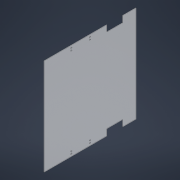
# Autodesk Inventor part: TopV5
Saved by Autodesk Inventor 2022 (Build 260153000, 153)
## iProperties
Created: 2021-10-02
Part Number: TopV5
Material: Acrylic, Clear
Document SubType Name: Sheet Metal
Designer: timmy
Density: 1.19 g/cm^3
Appearance: Transparent - Clear
Sheet Metal Rule: Default
Author: timmy
Autodesk Inventor part; units mm, degrees
ref_plane "YZ Plane" through (0, 0, 0) normal (1, 0, 0) x (0, 1, 0)
ref_plane "XZ Plane" through (0, 0, 0) normal (0, 1, 0) x (-1, 0, 0)
ref_plane "XY Plane" through (0, 0, 0) normal (0, 0, 1) x (1, 0, 0)
sketch "Sketch1" plane through (0, 0, 0) normal (1, 0, 0) x (0, 1, 0)
  line L0 (0, 0) -> (533.4, 0)
  line L1 (533.4, 0) -> (533.4, -508)
  line L2 (533.4, -508) -> (0, -508)
  line L3 (0, -508) -> (0, 0)
  dimension "d0" = 533.4
  dimension "d1" = 508
  constraints: 8 end point, 2 parallel, 1 horizontal, 1 perpendicular
  measures "d0" distance of L1.end L2.end
  measures "d1" distance of L0.end L1.end
extrude "Extrusion1" add sketch "Sketch1" along normal blind 1.5875
sketch "Sketch3" plane through (0, 0, 0) normal (-1, 0, 0) x (0, 0, 1)
  line L0 (-508, 0) -> (-508, 533.4) projected
  line L1 (0, 0) -> (-508, 0) projected
  circle A0 centre (-358.14, 12.7) radius 3.302
  circle A1 centre (-358.14, 25.4) radius 3.302
  circle A2 centre (-149.86, 12.7) radius 3.302
  circle A3 centre (-149.86, 25.4) radius 3.302
  circle A4 centre (-254, 12.7) radius 3.302
  circle A5 centre (-254, 25.4) radius 3.302
  circle A6 centre (-358.14, 508) radius 3.302
  circle A7 centre (-358.14, 520.7) radius 3.302
  circle A8 centre (-149.86, 508) radius 3.302
  circle A9 centre (-149.86, 520.7) radius 3.302
  circle A10 centre (-254, 508) radius 3.302
  circle A11 centre (-254, 520.7) radius 3.302
  constraints: 12 centre point
extrude "Extrusion5" cut sketch "Sketch3" against normal up to surface (1.5875 mm away) contours A0 | A1 | A2 | A3 | A4 | A5
sheet face with bend "Face1" sketch "Sketch1" thickness 3.048 toward (1, 0, 0) bend radius 3.048
bend "Bend1"
extrude "Cut1" cut sketch "Sketch3" against normal up to surface (3.048 mm away)
sketch "Sketch4" plane through (3.048, 0, 0) normal (1, 0, 0) x (0, 0, -1)
  line L0 (508, 533.4) -> (508, 0) projected
  line L1 (508, 266.7) -> (434.34, 266.7)
  line L2 (0, 0) -> (508, 0) projected
  line L3 (434.34, 0) -> (434.34, 34.925)
  line L4 (434.34, 0) -> (469.265, 0) construction
  line L5 (434.34, 34.925) -> (349.377, 34.925)
  line L6 (434.34, 17.4625) -> (346.202, 17.4625)
  line L7 (346.202, 0) -> (346.202, 31.75)
  line L8 (346.202, 31.75) -> (349.377, 34.925)
  line L9 (434.34, 533.4) -> (434.34, 498.475)
  line L10 (434.34, 498.475) -> (349.377, 498.475)
  line L11 (434.34, 515.9375) -> (346.202, 515.9375)
  line L12 (346.202, 533.4) -> (346.202, 501.65)
  line L13 (346.202, 501.65) -> (349.377, 498.475)
  line L14 (0, 533.4) -> (508, 533.4) projected
  line L15 (508, 0) -> (0, 0) projected
  dimension "d42" = 73.66
  dimension "d43" = 34.925
  dimension "d44" = 90
  dimension "d45" = 84.963
  dimension "d46" = 88.138
  dimension "d47" = 31.75
  constraints: 24 end point, 7 symmetric about line, 4 horizontal, 2 midpoint, 2 point on line, 2 vertical, 1 perpendicular
  measures "d42" distance of L1.start L1.end
  measures "d43" distance of L3.start L3.end
  measures "d44" angle of L4 L3
  measures "d45" distance of L3.end L5.end
  measures "d46" distance of L6.start L6.end
  measures "d47" distance of L7.start L7.end
extrude "Cut2" cut sketch "Sketch4" against normal blind 3.048
equation "\"d38\" = Thickness"
equation "\"d48\" = Thickness"
equation "\"d32\" = Thickness"
equation "\"d33\" = BendRadius"
equation "\"d34\" = BendReliefWidth"
equation "\"d36\" = MinimumRemnant"
equation "\"d35\" = BendReliefDepth"
equation "\"d37\" = TransitionRadius"
equation "\"BendRadius\" = Thickness"
equation "\"BendReliefWidth\" = Thickness"
equation "\"BendReliefDepth\" = 0.5 * Thickness"
equation "\"CornerReliefSize\" = 4 * Thickness"
equation "\"MinimumRemnant\" = 2 * Thickness"
equation "\"TransitionRadius\" = BendRadius"
equation "\"JacobiRadiusSize\" = BendRadius"
equation "\"GapSize\" = Thickness"
equation "\"Thickness\" = 3.048"
body "Solid1"
